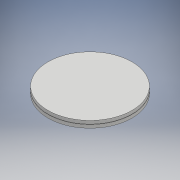
# Autodesk Inventor part: Game_CircleMarkers
Saved by Autodesk Inventor 2018 (Build 220112000, 112)
## iProperties
Created: 2021-04-21
Part Number: Game_CircleMarkers
Material: Generic
Document SubType Name: Modeling
Designer: Bradley
Density: 1 g/cm^3
Appearance: Default
Author: Bradley
Autodesk Inventor part; units mm, degrees
ref_plane "YZ Plane" through (0, 0, 0) normal (1, 0, 0) x (0, 1, 0)
ref_plane "XZ Plane" through (0, 0, 0) normal (0, 1, 0) x (-1, 0, 0)
ref_plane "XY Plane" through (0, 0, 0) normal (0, 0, 1) x (1, 0, 0)
sketch "Sketch1" plane through (0, 0, 0) normal (0, 0, 1) x (1, 0, 0)
  circle A0 centre (0, 0) radius 25
  dimension "d0" = 50
  constraints: 1 centre point, 1 coincident
  measures "d0" diameter of A0
extrude "Extrusion1" add sketch "Sketch1" along normal blind 1.9
pattern_linear "Rectangular Pattern1" count 2 spacing 2.1 along (0, 0, 1) of "Extrusion1"
body "Solid1"
